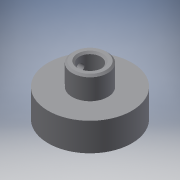
# Autodesk Inventor part: 齒輪
Saved by Autodesk Inventor 2016 SP1 (Build 200210100, 210)
## iProperties
Created: 2018-03-22
Part Number: 齒輪
Material: 一般
Document SubType Name: Modeling
Designer: admin
Density: 1 g/cm^3
Appearance: 預設
Author: admin
Autodesk Inventor part; units mm, degrees
ref_plane "YZ Plane" through (0, 0, 0) normal (1, 0, 0) x (0, 1, 0)
ref_plane "XZ Plane" through (0, 0, 0) normal (0, 1, 0) x (-1, 0, 0)
ref_plane "XY Plane" through (0, 0, 0) normal (0, 0, 1) x (1, 0, 0)
sketch "草圖1" plane through (0, 0, 0) normal (0, 0, 1) x (1, 0, 0)
  circle A0 centre (0, 0) radius 11.725
  dimension "d0" = 23.45
  constraints: 1 centre point, 1 coincident
  measures "d0" diameter of A0
extrude "擠出1" add sketch "草圖1" along normal blind 7.9
sketch "草圖2" plane through (0, 0, 7.9) normal (0, 0, 1) x (1, 0, 0)
  circle A0 centre (0, 0) radius 5
  dimension "d3" = 10
  constraints: 1 centre point, 1 coincident
  measures "d3" diameter of A0
extrude "擠出2" add sketch "草圖2" along normal blind 6.3
hole "孔1" at (0, 0, 14.2) direction (0, 0, -1) diameter 6 end through all
chamfer "倒角1" distance 0.5 angle 45 3 edges at (0, 3, 14.2) (0, 3, 0) (-5, 0, 14.2)
sketch "草圖3" plane through (0, 0, 0) normal (1, 0, 0) x (0, 1, 0)
  circle A0 centre (0, 10.9) radius 1.175
  line L0 (-4.5, 14.2) -> (4.5, 14.2) projected
  point P0 (0, 0)
  dimension "d18" = 2.35
  dimension "d19" = 3.3
  constraints: 1 centre point
  measures "d18" diameter of A0
  measures "d19" distance from line of L0 A0.centre
extrude "擠出3" cut sketch "草圖3" against normal through all
